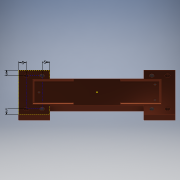
# Autodesk Inventor part: mount-base
Saved by Autodesk Inventor 2017 SP1 (Build 210196100, 196)
## iProperties
Created: 2017-02-03
Part Number: mount-base
Material: Copper
Document SubType Name: Modeling
Designer: Alex
Density: 8.94 g/cm^3
Appearance: Copper - Polished
Author: Alex
Autodesk Inventor part; units mm, degrees
ref_plane "YZ Plane" through (0, 0, 0) normal (1, 0, 0) x (0, 1, 0)
ref_plane "XZ Plane" through (0, 0, 0) normal (0, 1, 0) x (-1, 0, 0)
ref_plane "XY Plane" through (0, 0, 0) normal (0, 0, 1) x (1, 0, 0)
sketch "Sketch1" plane through (0, 0, 0) normal (0, 1, 0) x (-1, 0, 0)
  line L0 (-12, 30) -> (-12, -30)
  line L1 (12, -30) -> (12, 30)
  line L2 (20, 30) -> (12, 30)
  line L3 (-12, 30) -> (-20, 30)
  line L4 (-20, -30) -> (-12, -30)
  line L5 (12, -30) -> (20, -30)
  line L6 (20, 50) -> (-20, 50)
  line L7 (-20, -50) -> (20, -50)
  line L8 (20, -50) -> (20, -30)
  line L9 (20, 30) -> (20, 50)
  line L10 (-20, 50) -> (-20, 30)
  line L11 (-20, -30) -> (-20, -50)
  point P0 (0, 0)
  dimension "d21" = 100
  dimension "d22" = 60
  dimension "d23" = 40
  dimension "dw" = 8
  dimension "d25" = 8
  dimension "d26" = 8
  dimension "d27" = 8
  constraints: 24 end point, 10 parallel, 3 horizontal, 2 perpendicular
  measures "d21" distance between parallel lines of L7 L6
  measures "d22" distance between parallel lines of L4 L3
  measures "d23" distance between parallel lines of L11 L8
  measures "dw" distance between parallel lines of L1 L8
  measures "d25" distance between parallel lines of L9 L1
  measures "d26" distance between parallel lines of L0 L10
  measures "d27" distance between parallel lines of L0 L11
extrude "Extrusion1" add sketch "Sketch1" along normal blind 5
sketch "Sketch4" plane through (0, 5, 0) normal (0, 1, 0) x (1, 0, 0)
  line L0 (10, -40) -> (-10, -40)
  line L1 (-10, 40) -> (10, 40)
  line L2 (11, -41) -> (-11, -41)
  line L3 (-11, 41) -> (11, 41)
  line L4 (-11, -41) -> (-11, -15)
  line L5 (-11, 15) -> (-11, 41)
  line L6 (-10, -40) -> (-10, -15)
  line L7 (-10, 15) -> (-10, 40)
  line L8 (-11, -15) -> (-10, -15)
  line L9 (10, -15) -> (11, -15)
  line L10 (10, 40) -> (10, 15)
  line L11 (10, -15) -> (10, -40)
  line L12 (11, 41) -> (11, 15)
  line L13 (11, -15) -> (11, -41)
  line L14 (11, 15) -> (10, 15)
  line L15 (-10, 15) -> (-11, 15)
  point P0 (0, 0)
  dimension "d28" = 20
  dimension "d29" = 80
  dimension "d30" = 22
  dimension "d31" = 82
  constraints: 32 end point, 14 parallel, 4 horizontal, 4 perpendicular
  measures "d28" distance of L1.start L1.end
  measures "d29" distance of L0.end L1.start
  measures "d30" distance of L3.start L3.end
  measures "d31" distance of L2.end L3.start
extrude "Extrusion3" add sketch "Sketch4" along normal blind 1
fillet "Fillet3" radius 0.3 16 edges at (-11, 6, 28) (-10.5, 6, 15) (-10, 6, 27.5) (0, 6, 41) (0, 6, 40) (11, 6, 28) (10, 6, 27.5) (10.5, 6, 15) (10.5, 6, -15) (-10.5, 6, -15) (-11, 6, -28) (-10, 6, -27.5) (10, 6, -27.5) (11, 6, -28) (0, 6, -40) (0, 6, -41)
sketch "Sketch5" plane through (0, 5, 0) normal (0, 1, 0) x (1, 0, 0)
  line L0 (10, -40) -> (-10, -40) construction
  line L1 (-10, -40) -> (-10, 40) construction
  line L2 (-10, 40) -> (10, 40) construction
  line L3 (10, 40) -> (10, -40) construction
  line L4 (-7, -37) -> (7, -37) construction
  line L5 (7, -37) -> (7, 37) construction
  line L6 (7, 37) -> (-7, 37) construction
  line L7 (-7, 37) -> (-7, -37) construction
  line L8 (0, -37) -> (0, 37) construction
  point P0 (0, 0)
  dimension "baseH" = 20
  dimension "baseW" = 80
  dimension "d42" = 14
  dimension "d43" = 74
  constraints: 18 end point, 4 parallel, 2 horizontal, 2 midpoint, 2 perpendicular
  measures "baseH" distance of L1.end L2.end
  measures "baseW" distance of L0.end L1.end
  measures "d42" distance of L6.end L5.end
  measures "d43" distance of L5.end L4.end
hole "Hole2" at (0, 5, 37) at (-7, 5, -37) at (7, 5, -37) direction (0, -1, 0) diameter 1.567 end through all thread size "M2x0.4" class "6H" standard "ISO Metric profile"
sketch "Sketch6" plane through (0, 5, 0) normal (0, 1, 0) x (1, 0, 0)
  line L0 (-20, -30) -> (-20, -50) construction
  line L1 (-20, -50) -> (20, -50) construction
  line L2 (20, -50) -> (20, -30) construction
  line L3 (-15, -45) -> (15, -45) construction
  line L4 (15, -45) -> (15, -35) construction
  line L5 (15, -35) -> (-15, -35) construction
  line L6 (-15, -35) -> (-15, -45) construction
  line L7 (-12, -30) -> (-20, -30) construction
  line L8 (20, -30) -> (12, -30) construction
  point P0 (0, 0)
  dimension "d53" = 5
  dimension "d54" = 5
  dimension "d55" = 5
  dimension "d56" = 5
  constraints: 8 end point, 2 parallel, 1 horizontal, 1 perpendicular
  measures "d53" distance between parallel lines of L1 L3
  measures "d54" distance between parallel lines of L0 L6
  measures "d55" distance between parallel lines of L4 L2
  measures "d56" distance between parallel lines of L7 L5
hole "Hole4" at (-15, 5, 35) at (15, 5, 35) direction (0, -1, 0) diameter 3.242 end through all thread size "M4x0.7" class "6H" standard "ISO Metric profile"
hole "Hole5" at (-15, 5, 45) at (15, 5, 45) direction (0, -1, 0) diameter 3.4 end through all clearance for "Socket Head Cap Screw ISO 4762" size "M3" standard "ISO"
mirror "Mirror2" about plane through (0, 0, 0) normal (0, 0, 1) of "Hole4", "Hole5"
equation "\"d25\" = dw"
equation "\"d26\" = dw"
equation "\"d27\" = dw"
body "Solid1"
